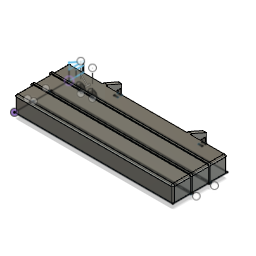
FuelTank (Autodesk Fusion 360 design; units mm, degrees)
Autodesk Fusion 360 part; units mm, degrees
note: some values were not read from the file. Set by a fixed rule: which sketch regions a step uses.
sketch "Sketch1" plane through (0, 0, 0) normal (0, 1, 0) x (1, 0, 0)
  line L0 (0, 0) -> (90, 0)
  line L1 (90, 0) -> (90, 31)
  line L2 (90, 31) -> (0, 31)
  line L3 (0, 31) -> (0, 0)
  line L4 (-3, 20.67) -> (93, 20.67) construction
  line L5 (-3, 10.33) -> (93, 10.33) construction
  line L6 (0, 21.17) -> (90, 21.17)
  line L7 (0, 20.17) -> (90, 20.17)
  line L8 (0, 9.83) -> (90, 9.83)
  line L9 (0, 10.83) -> (90, 10.83)
  line L10 (90, 20.17) -> (90.5, 20.17)
  line L11 (90.5, 20.17) -> (90.5, 21.17)
  line L12 (90.5, 21.17) -> (90, 21.17)
  line L13 (90, 21.17) -> (90, 20.17)
  line L14 (90, 10.83) -> (90.5, 10.83)
  line L15 (90.5, 10.83) -> (90.5, 9.83)
  line L16 (90.5, 9.83) -> (90, 9.83)
  line L17 (90, 9.83) -> (90, 10.83)
  line L18 (0, 21.17) -> (-0.5, 21.17)
  line L19 (-0.5, 21.17) -> (-0.5, 20.17)
  line L20 (-0.5, 20.17) -> (0, 20.17)
  line L21 (0, 20.17) -> (0, 21.17)
  line L22 (0, 9.83) -> (-0.5, 9.83)
  line L23 (-0.5, 9.83) -> (-0.5, 10.83)
  line L24 (-0.5, 10.83) -> (0, 10.83)
  line L25 (0, 10.83) -> (0, 9.83)
  line L26 (70, 39) -> (68, 39)
  line L27 (68, 39) -> (68, 38.5)
  line L28 (68, 38.5) -> (70, 38.5)
  line L29 (70, 38.5) -> (70, 39)
  line L30 (68, 37) -> (70, 37)
  line L31 (70, 37) -> (70, 36.5)
  line L32 (70, 36.5) -> (68, 36.5)
  line L33 (68, 36.5) -> (68, 37)
  line L34 (20, 37) -> (22, 37)
  line L35 (22, 37) -> (22, 36.5)
  line L36 (22, 36.5) -> (20, 36.5)
  line L37 (20, 36.5) -> (20, 37)
  line L38 (20, 38.5) -> (22, 38.5)
  line L39 (22, 38.5) -> (22, 39)
  line L40 (22, 39) -> (20, 39)
  line L41 (20, 39) -> (20, 38.5)
  dimension "d1" = 90
  dimension "d2" = 31
  dimension "d3" = 10.33
  dimension "d4" = 10.33
  dimension "d5" = 0.5
  dimension "d6" = 0.5
  dimension "d7" = 0.5
  dimension "d8" = 0.5
  dimension "d9" = 0.5
  dimension "d10" = 0.5
  dimension "d11" = 0.5
  dimension "d12" = 0.5
  dimension "d84" = 0.5
  dimension "d86" = 8
  dimension "d88" = 2
  dimension "d89" = 0.5
  dimension "d90" = 0.5
  dimension "d91" = 20
  dimension "d92" = 20
  dimension "d93" = 20
  dimension "d94" = 0.5
  dimension "d95" = 8
  dimension "d96" = 6
  dimension "d97" = 6
  constraint horizontal L0
  constraint vertical L1
  constraint horizontal L2
  constraint vertical L3
  constraint coincident L0.start L3.end
  constraint perpendicular L1 L4
  constraint perpendicular L3 L5
  constraint coincident L3 L6.start
  constraint coincident L1 L6.end
  constraint perpendicular L1 L6
  constraint coincident L3 L7.start
  constraint coincident L1 L7.end
  constraint perpendicular L1 L7
  constraint coincident L3 L8.start
  constraint coincident L1 L8.end
  constraint perpendicular L1 L8
  constraint coincident L1 L9.end
  constraint perpendicular L1 L9
  constraint horizontal L10
  constraint vertical L11
  constraint horizontal L12
  constraint vertical L13
  constraint horizontal L14
  constraint vertical L15
  constraint horizontal L16
  constraint vertical L17
  constraint horizontal L18
  constraint vertical L19
  constraint horizontal L20
  constraint vertical L21
  constraint horizontal L22
  constraint vertical L23
  constraint horizontal L24
  constraint vertical L25
  constraint horizontal L26
  constraint vertical L27
  constraint horizontal L28
  constraint vertical L29
  constraint horizontal L30
  constraint vertical L31
  constraint horizontal L32
  constraint vertical L33
  constraint horizontal L34
  constraint vertical L35
  constraint horizontal L36
  constraint vertical L37
  constraint horizontal L38
  constraint vertical L39
  constraint horizontal L40
  constraint vertical L41
  measures "d1" distance of L0.start L0.end
  measures "d2" distance of L0.start L2.end
  measures "d3" distance of L2 L4
  measures "d4" distance of L0 L5
  measures "d5" distance of L4 L6
  measures "d6" distance of L4 L7
  measures "d7" distance of L5 L9
  measures "d8" distance of L5 L8
  measures "d9" distance of L7.end L10.end
  measures "d10" distance of L9.end L14.end
  measures "d11" distance of L6.start L18.end
  measures "d12" distance of L8.start L22.end
  measures "d84" distance of L26.start L28.end
  measures "d86" distance of L2 L26.start
  measures "d88" distance of L27.end L28.end
  measures "d89" distance of L30.start L32.end
  measures "d90" distance of L34.start L36.end
  measures "d91" horizontal distance of L2.end L34.start
  measures "d92" horizontal distance of L1.end L26.start
  measures "d93" distance of L1 L30.end
  measures "d94" distance of L38.start L40.end
  measures "d95" distance of L2 L39.end
  measures "d96" distance of L2 L34
  measures "d97" distance of L2 L30
extrude "Extrude1" add sketch "Sketch1" along normal blind 9 contours L1 L2 L3 L6 makes body 1
extrude "Extrude2" add sketch "Sketch1" along normal blind 9 separate body contours L1 L3 L7 L9 makes body 2
extrude "Extrude3" add sketch "Sketch1" along normal blind 9 separate body contours L0 L1 L3 L8 makes body 3
extrude "Extrude4" add sketch "Sketch1" along normal blind 9.5 contours L1 L3 L6 L7 L13 L21 bodies 1 2
extrude "Extrude5" add sketch "Sketch1" along normal blind 9.5 contours L1 L3 L8 L9 L17 L25 bodies 1 3
extrude "Extrude6" add sketch "Sketch1" along normal blind 9.5 contours L1 L10 L11 L12 L13 bodies 1
extrude "Extrude7" add sketch "Sketch1" along normal blind 9.5 contours L1 L14 L15 L16 L17 bodies 1
extrude "Extrude8" add sketch "Sketch1" along normal blind 9.5 contours L3 L18 L19 L20 L21 bodies 1
extrude "Extrude9" add sketch "Sketch1" along normal blind 9.5 contours L3 L22 L23 L24 L25 bodies 1
sketch "Sketch2" plane through (0, 0, 0) normal (1, 0, 0) x (0, 0, -1)
  line L0 (39, 0) -> (31, 0)
  line L1 (31, 0) -> (31, 5.5)
  line L2 (31, 5.5) -> (39, 5.5)
  line L3 (39, 5.5) -> (39, 0)
  line L4 (31, 9) -> (39, 5.5)
  line L5 (31, 9) -> (31, 5.5)
  line L6 (39, 0) -> (35, 0)
  line L7 (35, 0) -> (35, 3.5)
  line L8 (35, 3.5) -> (39, 3.5)
  line L9 (39, 3.5) -> (39, 0)
  point P0 (31, 0)
  dimension "d33" = 8
  dimension "d34" = 8
  dimension "d35" = 5.5
  dimension "d36" = 3.5
  dimension "d37" = 4
  constraint horizontal L0
  constraint vertical L1
  constraint horizontal L2
  constraint vertical L3
  constraint horizontal L6
  constraint vertical L7
  constraint horizontal L8
  constraint vertical L9
  measures "d33" distance of L0.start P0
  measures "d34" distance of L1 L3
  measures "d35" distance of L0 L2
  measures "d36" distance of L6 L8
  measures "d37" distance of L7 L9
extrude "Extrude10" add sketch "Sketch2" along normal blind 2 from surface at 68 contours L0 L1 L2 L3 L7 L8 | L2 L4 L5 bodies 1
extrude "Extrude11" add sketch "Sketch2" along normal blind 2 from surface at 20 contours L0 L1 L2 L3 L7 L8 | L2 L4 L5 bodies 1
fillet "Fillet1" radius 1 1 edges at (90, 9, -4.915) on bodies 1
fillet "Fillet2" radius 1 1 edges at (90, 9, -15.5) on bodies 1
fillet "Fillet3" radius 1 1 edges at (90, 9, -26.085) on bodies 1
fillet "Fillet4" radius 1 3 edges at (90, 4, -31) (89.7071, 8.7071, -31) (79.5, 9, -31) on bodies 1
fillet "Fillet5" radius 1 3 edges at (90, 4, 0) (89.7071, 8.7071, 0) (44.5, 9, 0) on bodies 1
fillet "Fillet6" radius 1 3 edges at (0, 4, 0) (0, 8.7071, -0.2929) (0, 9, -5.415) on bodies 1
fillet "Fillet7" radius 1 1 edges at (0, 9, -15.5) on bodies 1
fillet "Fillet8" radius 1 1 edges at (0, 9, -26.085) on bodies 1
fillet "Fillet9" radius 1 3 edges at (0, 4, -31) (0.2929, 8.7071, -31) (10.5, 9, -31) on bodies 1
fillet "Fillet10" radius 1 1 edges at (45, 9, -31) on bodies 1
sketch "Sketch3" plane through (0, 0, -31) normal (0, 0, -1) x (-1, 0, 0)
  line L0 (-1, 8) -> (-20, 8)
  line L1 (-20, 8) -> (-20, 0)
  line L2 (-20, 0) -> (-1, 0)
  line L3 (-1, 0) -> (-1, 8)
  line L4 (-6.666, -3) -> (-6.666, 13) construction
  line L5 (-13.333, -2) -> (-13.333, 13) construction
  circle A0 centre (-6.666, 0) radius 2.5
  circle A1 centre (-13.333, 0) radius 2.5
  dimension "d64" = 6.667
  dimension "d65" = 6.667
  dimension "d66" = 5
  dimension "d67" = 5
  constraint perpendicular L2 L4
  constraint perpendicular L2 L5
  constraint coincident L4 A0.centre
  constraint coincident L2 A0.centre
  constraint coincident L5 A1.centre
  constraint coincident L2 A1.centre
  measures "d64" distance of L4 L5
  measures "d65" distance of L1 L5
  measures "d66" diameter of A0
  measures "d67" diameter of A1
extrude "Extrude12" add sketch "Sketch3" along normal blind 1.5 contours L2 A0 picked at (-6.0551, 0.5668) bodies 1
extrude "Extrude13" add sketch "Sketch3" along normal blind 1.5 contours L2 A1 picked at (-12.6445, 0.4694) bodies 1
fillet "Fillet11" radius 1 1 edges at (6.666, 2.5, -32.5) on bodies 1
fillet "Fillet12" radius 1 1 edges at (13.333, 2.5, -32.5) on bodies 1
fillet "Fillet13" radius 1 1 edges at (90.5, 9.5, -20.67) on bodies 1
fillet "Fillet14" radius 1 1 edges at (90.5, 9.5, -10.33) on bodies 1
fillet "Fillet15" radius 1 1 edges at (-0.5, 9.5, -20.67) on bodies 1
fillet "Fillet16" radius 1 1 edges at (-0.5, 9.5, -10.33) on bodies 1
extrude "Extrude14" add sketch "Sketch1" along normal blind 3.5 contours L26 L27 L28 L29 | L30 L31 L32 L33 bodies 1
extrude "Extrude15" add sketch "Sketch1" along normal blind 3.5 contours L34 L35 L36 L37 | L38 L39 L40 L41 bodies 1
